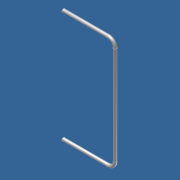
# Autodesk Inventor part: FE-00002-06
Saved by Autodesk Inventor 2012 (Build 160160000, 160)
## iProperties
Created: 2008-05-14
Part Number: FE-00002-06
Document SubType Name: Modeling
Designer: narosenberg
Density: 1 g/cm^3
Mass: 677.573 g
Surface Area: 4017.82 cm^2
Volume: 677.573 cm^3
Material: Default
Author: narosenberg
Autodesk Inventor part; units mm, degrees
ref_plane "XZ Plane" through (0, 0, 0) normal (0, 1, 0) x (-1, 0, 0)
ref_plane "XY Plane" through (0, 0, 0) normal (0, 0, 1) x (1, 0, 0)
sketch "Sketch1" plane through (0, 0, 0) normal (0, 0, 1) x (1, 0, 0)
  line L0 (-573.2124, 986.9902) -> (-116.0124, 986.9902)
  line L1 (-48.5119, 919.4897) -> (-48.5119, -80.5718)
  line L2 (-116.0124, -148.0723) -> (-573.2124, -148.0723)
  arc A0 (-48.5119, 919.4897) -> (-116.0124, 986.9902) centre (-116.0124, 919.4897) ccw
  arc A1 (-116.0124, -148.0723) -> (-48.5119, -80.5718) centre (-116.0124, -80.5718) ccw
  dimension "d2" = 67.5005
  dimension "d3" = 67.5005
  dimension "d4" = 1135.0625
  dimension "d5" = 524.7005
  constraints: 6 end point, 4 point on circle, 4 tangent, 2 centre point, 2 perpendicular, 1 horizontal, 1 vertical alignment
  measures "d2" radius of A0
  measures "d3" radius of A1
  measures "d4" distance between parallel lines of L2 L0
  measures "d5" distance from line of L0.start L1
ref_plane "Work Plane1" through (-573.2124, 986.9902, 0) normal (1, 0, 0) x (0, 1, 0)
sketch "Sketch2" plane through (-573.2124, 986.9902, 0) normal (1, 0, 0) x (0, 1, 0)
  circle A0 centre (0, 0) radius 16.7005
  dimension "d6" = 33.401
  constraints: 1 centre point
  measures "d6" diameter of A0
sweep "Sweep1" add profiles "Sketch2" path "Sketch1" path curves L0 A0 L1 A1 L2
shell "Shell1" thickness 3.3782 removed faces 2 at (-573.2124, 983.778, 7.5643) at (-573.2124, -144.9099, -4.5814)
equation "\"d3\" = d2"
body "Solid1"
